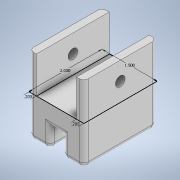
# Autodesk Inventor part: Sample Holder end for 8020-valveholder
Saved by Autodesk Inventor 2020 (Build 240168000, 168)
## iProperties
Created: 2022-02-15
Part Number: Sample Holder end for 8020-valveholder
Material: Generic
Document SubType Name: Modeling
Designer: Beaucage
Density: 1 g/cm^3
Appearance: Default
Author: Beaucage
Autodesk Inventor part; units mm, degrees
ref_plane "YZ Plane" through (0, 0, 0) normal (1, 0, 0) x (0, 1, 0)
ref_plane "XZ Plane" through (0, 0, 0) normal (0, 1, 0) x (-1, 0, 0)
ref_plane "XY Plane" through (0, 0, 0) normal (0, 0, 1) x (1, 0, 0)
sketch "Sketch1" plane through (0, 0, 0) normal (0, 1, 0) x (-1, 0, 0)
  line L0 (0, 0) -> (38.1, 0)
  line L1 (38.1, 0) -> (38.1, -50.8)
  line L2 (38.1, -50.8) -> (0, -50.8)
  line L3 (0, -50.8) -> (0, 0)
  line L4 (38.1, -50.8) -> (33.02, -50.8)
  line L5 (33.02, -50.8) -> (33.02, 0)
  line L6 (33.02, 0) -> (38.1, 0)
  line L7 (38.1, 0) -> (38.1, -50.8)
  line L8 (0, -50.8) -> (5.08, -50.8)
  line L9 (5.08, -50.8) -> (5.08, 0)
  line L10 (5.08, 0) -> (0, 0)
  line L11 (0, 0) -> (0, -50.8)
  dimension "d0" = 38.1
  dimension "d1" = 50.8
  dimension "d2" = 5.08
  dimension "d3" = 5.08
  constraints: 24 end point, 6 parallel, 3 horizontal, 3 perpendicular, 2 point on line
  measures "d0" distance of L1.end L2.end
  measures "d1" distance of L0.end L1.end
  measures "d2" distance of L5.end L6.end
  measures "d3" distance of L10.end L9.end
extrude "Extrusion1" add sketch "Sketch1" along normal blind 25.4 contours L0 L9 L2 L3 | L0 L1 L2 L5
extrude "Extrusion2" add sketch "Sketch1" against normal blind 13.97
sketch "Sketch2" plane through (0, 25.4, 0) normal (1, 0, 0) x (0, 0, -1)
  line L0 (50.8, 0) -> (0, 0) projected
  line L1 (25.4, 0) -> (25.4, -12.7)
  point P0 (0, -25.4)
  dimension "d8" = 12.7
  constraints: 2 end point, 1 midpoint, 1 vertical
  measures "d8" distance of L1.start L1.end
hole "Hole1" at (0, 12.7, -25.4) direction (-1, 0, 0) diameter 6.7564 end through all clearance for "Socket Head Cap Screw" size "1/4" standard "Ansi Unified Screw Threads"
sketch "Sketch3" plane through (0, -13.97, 0) normal (0, -1, 0) x (1, 0, 0)
  line L0 (-38.1, -28.7782) -> (-38.1, -22.0218) projected
  line L1 (-38.1, -25.4) -> (-19.05, -25.4)
  line L2 (0, 0) -> (-38.1, 0) projected
  line L3 (-14.605, -50.8) -> (-23.495, -50.8)
  line L4 (-23.495, -50.8) -> (-23.495, 0)
  line L5 (-23.495, 0) -> (-14.605, 0)
  line L6 (-14.605, 0) -> (-14.605, -50.8)
  line L7 (-14.605, -50.8) -> (-23.495, 0) construction
  line L8 (-23.495, -50.8) -> (-14.605, 0) construction
  circle A0 centre (-19.05, -25.4) radius 9.906
  line L9 (-38.1, -50.8) -> (0, -50.8)
  line L10 (0, -50.8) -> (0, 0)
  line L11 (0, 0) -> (-38.1, 0)
  line L12 (-38.1, 0) -> (-38.1, -50.8)
  line L13 (-38.1, -50.8) -> (0, 0) construction
  line L14 (0, -50.8) -> (-38.1, 0) construction
  point P0 (-14.605, -16.5473)
  point P1 (-14.605, -34.2527)
  point P2 (-23.495, -34.2527)
  point P3 (-23.495, -16.5473)
  dimension "d16" = 19.05
  dimension "d17" = 8.89
  dimension "d18" = 19.812
  constraints: 26 end point, 5 midpoint, 4 parallel, 3 horizontal, 2 perpendicular, 1 centre point, 1 coincident, 1 point on line
  measures "d16" distance of L1.start L1.end
  measures "d17" distance of L4.end L5.end
  measures "d18" diameter of A0
extrude "Extrusion3" add sketch "Sketch3" along normal blind 13.97 contours L0 L1 A0 L4 L9 L12 | L0 L12 L2 L4 A0 L1 | L6 A0 L2 L10 L9
fillet "Fillet1" radius 3.175 14 edges at (-38.1, -1.27, -50.8) (0, -1.27, -50.8) (-7.3025, -27.94, -50.8) (0, -27.94, -25.4) (-30.7975, -27.94, -50.8) (-7.3025, -27.94, 0) (-30.7975, -27.94, 0) (-38.1, -27.94, -25.4) (-38.1, -1.27, 0) (0, -1.27, 0) (-14.605, -27.94, -42.5264) (-14.605, -27.94, -8.2736) (-23.495, -27.94, -8.2736) (-23.495, -27.94, -42.5264)
fillet "Fillet2" radius 3.175 14 edges at (-19.05, -13.97, 0) (-19.05, -13.97, -50.8) (-24.4249, -27.0101, -0.9299) (-23.495, -19.3675, 0) (-13.6751, -27.0101, -0.9299) (-14.605, -19.3675, 0) (-13.6751, -27.0101, -49.8701) (-7.3025, -27.94, -47.625) (-3.175, -27.0101, -49.8701) (-14.605, -19.3675, -50.8) (-34.925, -27.0101, -49.8701) (-30.7975, -27.94, -47.625) (-24.4249, -27.0101, -49.8701) (-23.495, -19.3675, -50.8)
body "Solid1"
